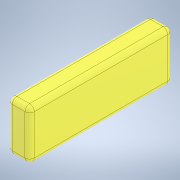
# Autodesk Inventor part: LiPo3S1P
Saved by Autodesk Inventor 2020.3 (Build 243373000, 373)
## iProperties
Created: 2021-04-22
Part Number: LiPo3S1P
Material: Nylon 6/6
Document SubType Name: Modeling
Designer: alexo
Density: 1.13 g/cm^3
Appearance: Smooth - Yellow
Author: alexo
Autodesk Inventor part; units mm, degrees
ref_plane "YZ Plane" through (0, 0, 0) normal (1, 0, 0) x (0, 1, 0)
ref_plane "XZ Plane" through (0, 0, 0) normal (0, 1, 0) x (-1, 0, 0)
ref_plane "XY Plane" through (0, 0, 0) normal (0, 0, 1) x (1, 0, 0)
sketch "Sketch1" plane through (0, 0, 0) normal (0, 1, 0) x (-1, 0, 0)
  line L0 (-10, -65) -> (10, -65)
  line L1 (10, -65) -> (10, 65)
  line L2 (10, 65) -> (-10, 65)
  line L3 (-10, 65) -> (-10, -65)
  line L4 (-10, -65) -> (10, 65) construction
  line L5 (10, -65) -> (-10, 65) construction
  point P0 (0, 0)
  dimension "d0" = 20
  dimension "d1" = 130
  constraints: 12 end point, 2 midpoint, 2 parallel, 1 horizontal, 1 perpendicular
  measures "d0" distance of L1.end L2.end
  measures "d1" distance of L0.end L1.end
extrude "Extrusion1" add sketch "Sketch1" along normal blind 45
fillet "Fillet1" radius 4.25 12 edges at (0, 0, -65) (-10, 22.5, -65) (0, 45, -65) (10, 22.5, -65) (10, 0, 0) (10, 45, 0) (10, 22.5, 65) (0, 0, 65) (0, 45, 65) (-10, 22.5, 65) (-10, 0, 0) (-10, 45, 0)
body "Solid1"
